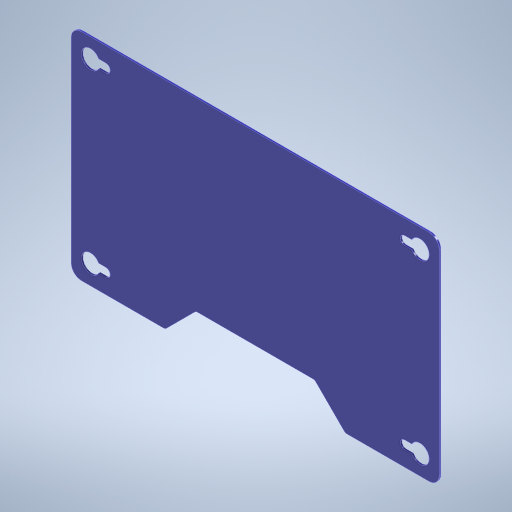
# Autodesk Inventor part: TorsoBackColorMarker
Saved by Autodesk Inventor 2024.2 (Build 282272000, 272)
## iProperties
Created: 2024-01-22
Part Number: TorsoBackColorMarker
Material: Polypropylene
Document SubType Name: Modeling
Designer: Masato Kubotera
Density: 0.899 g/cm^3
Appearance: Smooth - Navy
Mass: 16.5888 g
Surface Area: 500.852 cm^2
Volume: 18.4525 cm^3
Author: Masato Kubotera
Autodesk Inventor part; units mm, degrees
ref_plane "YZ Plane" through (0, 0, 0) normal (1, 0, 0) x (0, 1, 0)
ref_plane "XZ Plane" through (0, 0, 0) normal (0, 1, 0) x (-1, 0, 0)
ref_plane "XY Plane" through (0, 0, 0) normal (0, 0, 1) x (1, 0, 0)
derived "TorsoElectronicBoxBackFrame.ipt"
sketch "Sketch3" plane through (0, 0, 0) normal (1, 0, 0) x (0, 1, 0)
  line L0 (-90, 74.5) -> (90, 74.5) projected
  line L1 (0, 74.5) -> (0, -74.5) projected
  line L2 (90, 74.5) -> (90, -74.5) projected
  line L3 (90, -31) -> (-90, -31) projected
  arc A0 (76.5201, -23.6) -> (76.5201, -19.4) centre (80.5, -21.5) ccw projected
  line L4 (73, -23.6) -> (76.5201, -23.6) projected
  line L5 (73, -19.4) -> (76.5201, -19.4) projected
  arc A1 (73, -19.4) -> (73, -23.6) centre (73, -21.5) ccw projected
  arc A2 (76.5201, 62.9) -> (76.5201, 67.1) centre (80.5, 65) ccw projected
  line L6 (73, 62.9) -> (76.5201, 62.9) projected
  line L7 (73, 67.1) -> (76.5201, 67.1) projected
  arc A3 (73, 67.1) -> (73, 62.9) centre (73, 65) ccw projected
  line L8 (29, -16) -> (0, -16) projected
  line L9 (29, -16) -> (44, -31) projected
  point P0 (0, 0)
  point P1 (0, -31)
  point P2 (44.2, -31)
extrude "Extrusion1" add sketch "Sketch3" against normal blind 0.75 contours L0 L2 L3 L9 L8 L1
fillet "R5" radius 5 2 edges at (-0.375, 90, 74.5) (-0.375, 90, -31)
fillet "R2" radius 2 2 edges at (-0.375, 29, -16) (-0.375, 44, -31)
mirror "Mirror1" about plane through (0, 0, 0) normal (0, 1, 0)
sketch "Sketch1" plane through (0, 0, 0) normal (1, 0, 0) x (0, 1, 0)
  line L0 (-90, 74.5) -> (90, 74.5) projected
  line L1 (90, 74.5) -> (90, -74.5) projected
  line L2 (90, -74.5) -> (-90, -74.5) projected
  line L3 (-90, -74.5) -> (-90, 74.5) construction
  line L4 (-90, 74.5) -> (90, -74.5) construction
  line L5 (90, 74.5) -> (-90, -74.5) construction
  line L6 (85, 74.5) -> (85, 46.75) projected
  line L7 (85, 46.75) -> (90, 46.75) projected
  line L8 (0, 74.5) -> (0, -74.5) projected
  line L9 (90, 0) -> (-90, 0) construction
  arc A0 (85, 49.75) -> (85, 46.75) centre (85, 48.25) ccw projected
  line L10 (-90, 74.5) -> (-90, -74.5) projected
  circle A1 centre (73, 65) radius 3 construction
  arc A2 (73, 67.1) -> (73, 62.9) centre (73, 65) ccw construction
  line L11 (73, 67.1) -> (76.5201, 67.1) construction
  arc A3 (76.5201, 62.9) -> (76.5201, 67.1) centre (80.5, 65) ccw construction
  line L12 (73, 65) -> (80.5, 65) construction
  line L13 (73, 62.9) -> (76.5201, 62.9) construction
  line L14 (90, 28.75) -> (85, 28.75) construction
  line L15 (90, 14.75) -> (85, 14.75) construction
  line L16 (90, 21.75) -> (85, 21.75) construction
  line L17 (85, -3.25) -> (90, -3.25) projected
  arc A4 (85, -3.25) -> (85, -6.25) centre (85, -4.75) ccw projected
  line L18 (85, -6.25) -> (85, -74.5) projected
  line L19 (90, -31) -> (-90, -31) projected
  line L20 (74, -31) -> (74, -74.5) projected
  line L21 (-90, 21.75) -> (90, 21.75) construction
  circle A5 centre (73, -21.5) radius 3 construction
  arc A6 (73, -19.4) -> (73, -23.6) centre (73, -21.5) ccw construction
  line L22 (73, -23.6) -> (76.5201, -23.6) construction
  arc A7 (76.5201, -23.6) -> (76.5201, -19.4) centre (80.5, -21.5) ccw construction
  line L23 (73, -21.5) -> (80.5, -21.5) construction
  line L24 (73, -19.4) -> (76.5201, -19.4) construction
  arc A8 (74, -31) -> (74, -34) centre (74, -32.5) ccw projected
  point P0 (0, 0)
  point P1 (85, 65)
  point P2 (85, -21.5)
  constraints: 1 other
sketch "Sketch2" plane through (0, 0, 0) normal (1, 0, 0) x (0, 1, 0)
  line L0 (84.5, 34.25) -> (79.5, 34.25) construction
  line L1 (79.5, 34.25) -> (79.5, 9.25) construction
  line L2 (79.5, 9.25) -> (84.5, 9.25) construction
  line L3 (84.5, 9.25) -> (84.5, 34.25) construction
  line L4 (84.5, 34.25) -> (79.5, 9.25) construction
  line L5 (79.5, 34.25) -> (84.5, 9.25) construction
  line L6 (84.55, 34.3) -> (79.45, 34.3) projected
  line L7 (79.45, 34.3) -> (79.45, 9.2) projected
  line L8 (79.45, 9.2) -> (84.55, 9.2) projected
  line L9 (84.55, 9.2) -> (84.55, 34.3) projected
  line L10 (84.55, 34.3) -> (79.45, 9.2) construction
  line L11 (79.45, 34.3) -> (84.55, 9.2) construction
  arc A0 (84.55, 31.3) -> (84.55, 34.3) centre (84.55, 32.8) ccw projected
  line L12 (82, 34.25) -> (82, 9.25) construction
  arc A1 (79.45, 34.3) -> (79.45, 31.3) centre (79.45, 32.8) ccw projected
  line L13 (-90, 21.75) -> (90, 21.75) construction
  line L14 (0, 74.5) -> (0, -74.5) projected
  arc A2 (84.55, 9.2) -> (84.55, 12.2) centre (84.55, 10.7) ccw projected
  arc A3 (79.45, 12.2) -> (79.45, 9.2) centre (79.45, 10.7) ccw projected
  line L15 (-90, 74.5) -> (90, 74.5) projected
  line L16 (75.8, 74.5) -> (75.8, 69.5) projected
  line L17 (60.75, 69.5) -> (60.75, 74.5) construction
  line L18 (75.8, 69.5) -> (60.7, 69.5) projected
  line L19 (60.7, 69.5) -> (60.7, 74.5) projected
  line L20 (75.75, 69.5) -> (75.75, 74.5) construction
  line L21 (75.75, 69.5) -> (60.75, 69.5) construction
  line L22 (68.25, 69.5) -> (68.25, 74.5) construction
  arc A4 (73.6787, 69.5) -> (75.8, 71.6213) centre (74.7393, 70.5607) ccw projected
  arc A5 (60.7, 71.6213) -> (62.8213, 69.5) centre (61.7607, 70.5607) ccw projected
  line L23 (90, 74.5) -> (90, -74.5) projected
  line L24 (51.5, 59) -> (75.45, 59) projected
  line L25 (75.45, 59) -> (75.45, -0.5) projected
  line L26 (75.45, -0.5) -> (51.5, -0.5) projected
  line L27 (51.5, -0.5) -> (51.5, 59) projected
  line L28 (51.5, 59) -> (75.45, -0.5) construction
  line L29 (75.45, 59) -> (51.5, -0.5) construction
  line L30 (66.5, 67) -> (51.5, 67) construction
  line L31 (51.5, 67) -> (51.5, 62) construction
  line L32 (51.5, 62) -> (66.5, 62) construction
  line L33 (66.5, 62) -> (66.5, 67) construction
  line L34 (66.5, 67) -> (51.5, 62) construction
  line L35 (51.5, 67) -> (66.5, 62) construction
  line L36 (57.5, 67) -> (57.5, 62) construction
  line L37 (54.5, 67) -> (54.5, 62) construction
  line L38 (66.5, 64.5) -> (51.5, 64.5) construction
  line L39 (51.45, 67.05) -> (57.55, 67.05) projected
  line L40 (57.55, 67.05) -> (57.55, 61.95) projected
  line L41 (57.55, 61.95) -> (51.45, 61.95) projected
  line L42 (51.45, 61.95) -> (51.45, 67.05) projected
  line L43 (51.45, 67.05) -> (57.55, 61.95) construction
  line L44 (57.55, 67.05) -> (51.45, 61.95) construction
  arc A6 (57.55, 67.05) -> (54.55, 67.05) centre (56.05, 67.05) ccw projected
  arc A7 (53.5713, 67.05) -> (51.45, 64.9287) centre (52.5107, 65.9893) ccw projected
  arc A8 (54.55, 61.95) -> (57.55, 61.95) centre (56.05, 61.95) ccw projected
  arc A9 (51.45, 64.0713) -> (53.5713, 61.95) centre (52.5107, 63.0107) ccw projected
  line L45 (-51.5, -16) -> (51.5, -16) construction
  line L46 (51.5, -16) -> (51.5, 74.5) construction
  line L47 (51.5, 74.5) -> (-51.5, 74.5) construction
  line L48 (-51.5, 74.5) -> (-51.5, -16) construction
  line L49 (-51.5, -16) -> (51.5, 74.5) construction
  line L50 (51.5, -16) -> (-51.5, 74.5) construction
  line L51 (85, 74.5) -> (-85, 74.5) construction
  line L52 (75.45, 29.25) -> (51.5, 29.25) construction
  circle A10 centre (62.5, 64.5) radius 2.75 construction
  circle A11 centre (62.5, 64.5) radius 3.25 construction
  line L53 (57.55, -3.45) -> (51.45, -3.45) projected
  line L54 (57.55, -8.55) -> (57.55, -3.45) projected
  line L55 (51.45, -8.55) -> (57.55, -3.45) construction
  arc A12 (51.45, -6.4287) -> (53.5713, -8.55) centre (52.5107, -7.4893) ccw projected
  arc A13 (54.55, -8.55) -> (57.55, -8.55) centre (56.05, -8.55) ccw projected
  circle A14 centre (62.5, -6) radius 2.75 construction
  line L56 (66.5, -3.5) -> (66.5, -8.5) construction
  circle A15 centre (62.5, -6) radius 3.25 construction
  arc A16 (57.55, -3.45) -> (54.55, -3.45) centre (56.05, -3.45) ccw projected
  line L57 (66.5, -8.5) -> (51.5, -8.5) construction
  line L58 (66.5, -8.5) -> (51.5, -3.5) construction
  line L59 (51.5, -3.5) -> (66.5, -3.5) construction
  line L60 (66.5, -6) -> (51.5, -6) construction
  line L61 (51.5, -8.5) -> (66.5, -3.5) construction
  arc A17 (53.5713, -3.45) -> (51.45, -5.5713) centre (52.5107, -4.5107) ccw projected
  line L62 (51.5, -8.5) -> (51.5, -3.5) construction
  line L63 (57.5, -8.5) -> (57.5, -3.5) construction
  line L64 (54.5, -8.5) -> (54.5, -3.5) construction
  line L65 (51.45, -8.55) -> (57.55, -8.55) projected
  line L66 (51.45, -3.45) -> (51.45, -8.55) projected
  line L67 (57.55, -8.55) -> (51.45, -3.45) construction
  line L68 (90, -74.5) -> (-90, -74.5) projected
  line L69 (-90, 74.5) -> (-90, -74.5) projected
  line L70 (90, -31) -> (-90, -31) projected
  line L71 (49.2, -16) -> (44.2, -16) construction
  line L72 (44.2, -16) -> (44.2, -31) construction
  line L73 (44.2, -31) -> (49.2, -31) construction
  line L74 (49.2, -31) -> (49.2, -16) construction
  line L75 (49.2, -16) -> (44.2, -31) construction
  line L76 (44.2, -16) -> (49.2, -31) construction
  line L77 (49.2, -22) -> (44.2, -22) construction
  line L78 (49.2, -19) -> (44.2, -19) construction
  line L79 (46.7, -16) -> (46.7, -31) construction
  line L80 (44.15, -15.95) -> (49.25, -15.95) projected
  line L81 (49.25, -15.95) -> (49.25, -22.05) projected
  line L82 (49.25, -22.05) -> (44.15, -22.05) projected
  line L83 (44.15, -22.05) -> (44.15, -15.95) projected
  line L84 (44.15, -15.95) -> (49.25, -22.05) construction
  line L85 (49.25, -15.95) -> (44.15, -22.05) construction
  arc A18 (49.25, -22.05) -> (49.25, -19.05) centre (49.25, -20.55) ccw projected
  arc A19 (49.25, -18.0713) -> (47.1287, -15.95) centre (48.1893, -17.0107) ccw projected
  arc A20 (46.2713, -15.95) -> (44.15, -18.0713) centre (45.2107, -17.0107) ccw projected
  arc A21 (44.15, -19.05) -> (44.15, -22.05) centre (44.15, -20.55) ccw projected
  line L86 (-46.5, -11) -> (46.5, -11) projected
  line L87 (46.5, -11) -> (46.5, 69.5) projected
  line L88 (46.5, 69.5) -> (-46.5, 69.5) projected
  line L89 (-46.5, 69.5) -> (-46.5, -11) projected
  line L90 (-46.5, -11) -> (46.5, 69.5) construction
  line L91 (46.5, -11) -> (-46.5, 69.5) construction
  line L92 (29, -16) -> (0, -16) projected
  line L93 (29, -16) -> (44, -31) projected
  point P0 (0, 0)
  point P1 (82, 21.75)
  point P2 (82, 21.75)
  point P3 (63.475, 29.25)
  point P4 (59, 64.5)
  point P5 (54.5, 64.5)
  point P6 (0, 29.25)
  point P7 (59, -6)
  point P8 (54.5, -6)
  point P9 (77.95, 32.8)
  point P10 (46.7, -23.5)
  point P11 (46.7, -27)
  point P12 (46.7, -19)
  point P13 (0, 29.25)
  point P14 (44.2, -31)
  point P15 (0, -31)
  point P16 (82, 40.25)
  point P17 (82, 3.25)
  constraints: 1 other
body "Solid4"
